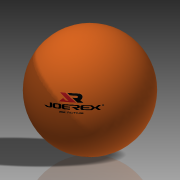
# Autodesk Inventor part: Joerex TT ball
Saved by Autodesk Inventor 2013 (Build 170138000, 138)
## iProperties
Created: 2014-03-24
Part Number: Joerex TT ball
Material: PVC, Unplasticized
Document SubType Name: Modeling
Designer: Nahid Mubin
Density: 1 g/cm^3
Author: Nahid Mubin
Autodesk Inventor part; units mm, degrees
ref_plane "YZ Plane" through (0, 0, 0) normal (1, 0, 0) x (0, 1, 0)
ref_plane "XZ Plane" through (0, 0, 0) normal (0, 1, 0) x (-1, 0, 0)
sketch "Sketch1" plane through (0, 0, 0) normal (0, 0, 1) x (1, 0, 0)
  arc A0 (0, 20) -> (0, -20) centre (0, 0) ccw
  arc A1 (0, 19) -> (0, -19) centre (0, 0) ccw
  line L0 (0, -20) -> (0, 20)
  dimension "d0" = 40
  dimension "d1" = 1
  constraints: 4 point on circle, 2 centre point, 2 end point, 2 point on line, 1 coincident, 1 vertical
  measures "d0" diameter of A0
  measures "d1" radial gap between concentric circles of A0 A1
revolve "Revolution1" add sketch "Sketch1" angle 360 about axis through (0, -20, 0) along (0, 1, 0) contours L0 A1 A0
ref_plane "Work Plane2" through (0, 0, 36.25) normal (0, 0, 1) x (1, 0, 0)
sketch "Sketch5" plane through (0, 0, 36.25) normal (0, 0, 1) x (1, 0, 0)
  line L0 (-10, 3.5833) -> (10, 3.5833) construction
  line L1 (10, 3.5833) -> (10, -3.5833) construction
  line L2 (10, -3.5833) -> (-10, -3.5833) construction
  line L3 (-10, -3.5833) -> (-10, 3.5833) construction
  circle A0 centre (0, 0) radius 20 projected
  dimension "d22" = 20
  dimension "d27" = 7.1667
  dimension "d30" = 10
  dimension "d31" = 3.5833
  constraints: 2 other
  measures "d22" distance of L0.start L0.end
  measures "d27" distance of L2.end L0.start
  measures "d30" distance from line of A0.centre L1
  measures "d31" distance from line of A0.centre L2
decal "Decal2"
equation "\"d30\" = 0.5 * d22"
equation "\"d31\" = 0.5 * d27"
body "Solid1"
